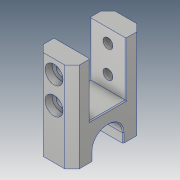
# Autodesk Inventor part: 200-50-WHEEL-CONNECTOR-20MM-01
Saved by Autodesk Inventor 2018.2 (Build 222227000, 227)
## iProperties
Manager: feesmrt
Company: FRANC0R
Created: 2017-12-05
Part Number: 200-50-WHEEL-CONNECTOR-20MM-01
Material: Aluminium 6061
Document SubType Name: Modeling
Designer: feesmrt
Density: 2.7 g/cm^3
Appearance: Aluminium - flach
Project: Rescue Robot
Cost Center: -
Engineer: feesmrt
Authority: feesmrt
Description: Wheel Connector 20mm Part 1
Stock Number: 200-50-WHEEL-CONNECTOR-20MM-01
Author: feesmrt
Subject: Rescue Robot
Title: Wheel Connector 20mm Part 1
Revision Number: 1
Autodesk Inventor part; units mm, degrees
note: some values were not read from the file. Chosen so that the rebuilt part matches the saved one: direction of "DIN7984_M5_Boh".
ref_plane "YZ Plane" through (0, 0, 0) normal (1, 0, 0) x (0, 1, 0)
ref_plane "XZ Plane" through (0, 0, 0) normal (0, 1, 0) x (-1, 0, 0)
ref_plane "XY Plane" through (0, 0, 0) normal (0, 0, 1) x (1, 0, 0)
sketch "Skizze1" plane through (0, 0, 0) normal (1, 0, 0) x (0, 1, 0)
  line L0 (-28, 0) -> (28, 0) construction
  line L1 (0, 35) -> (0, -35) construction
  line L2 (-20, -25) -> (20, -25)
  line L3 (20, -25) -> (20, 25)
  line L4 (20, 25) -> (-20, 25)
  line L5 (-20, 25) -> (-20, -25)
  line L6 (-20, -25) -> (20, 25) construction
  line L7 (20, -25) -> (-20, 25) construction
  point P0 (0, 0)
  dimension "d0" = 40
  dimension "d1" = 50
  constraints: 12 end point, 2 midpoint, 2 parallel, 1 horizontal, 1 perpendicular
  measures "d0" distance of L3.end L4.end
  measures "d1" distance of L2.end L3.end
extrude "Grundkörper" add sketch "Skizze1" along normal mid plane 20
sketch "Skizze2" plane through (10, 0, 0) normal (1, 0, 0) x (0, 0, -1)
  line L0 (-25, 20) -> (-25, -20) construction
  line L1 (0, -28) -> (0, 28) construction
  line L2 (-35, 0) -> (35, 0) construction
  line L3 (-25, -10) -> (5, -10)
  line L4 (5, -10) -> (5, 10)
  line L5 (5, 10) -> (-25, 10)
  line L6 (-25, 10) -> (-25, -10)
  line L7 (25, -20) -> (25, 20) construction
  line L8 (25, -8.4) -> (20, -8.4)
  line L9 (12, -0.4) -> (12, 0.4)
  line L10 (20, 8.4) -> (25, 8.4)
  line L11 (25, -8.4) -> (25, 8.4)
  arc A0 (12, -0.4) -> (20, -8.4) centre (20, -0.4) ccw
  arc A1 (20, 8.4) -> (12, 0.4) centre (20, 0.4) ccw
  point P0 (0, 0)
  dimension "d4" = 30
  dimension "d5" = 20
  dimension "d14" = 13
  dimension "d15" = 16.8
  dimension "d16" = 8
  constraints: 16 end point, 4 perpendicular, 4 point on circle, 4 tangent, 3 point on line, 2 centre point, 2 horizontal, 2 parallel, 1 equal radius, 2 other
  measures "d4" distance of L3.start L3.end
  measures "d5" distance between parallel lines of L5 L3
  measures "d14" distance between parallel lines of L7 L9
  measures "d15" distance between parallel lines of L8 L10
  measures "d16" radius of A0
extrude "Ausschnitt" cut sketch "Skizze2" against normal through all
sketch "Skizze4" plane through (-10, -20, -25) normal (0, -1, 0) x (1, 0, 0)
  line L0 (20, 20) -> (0, 20) construction
  line L1 (20, 50) -> (0, 50) construction
  line L2 (10, 60) -> (10, -10) projected
  line L3 (0, 35) -> (20, 35) construction
  line L4 (0, 0) -> (0, 50) construction
  line L5 (20, 50) -> (20, 0) construction
  point P0 (10, 25)
  point P1 (10, 42.5)
  point P2 (10, 27.5)
  dimension "d19" = 30
  dimension "d20" = 15
  dimension "d21" = 15
  constraints: 4 point on line, 2 end point, 1 horizontal, 1 symmetric about line
  measures "d19" distance between parallel lines of L0 L1
  measures "d20" distance between parallel lines of L1 L3
  measures "d21" distance of point (10, 27.5) point (10, 42.5)
hole "DIN7984_M5_Boh" at (0, -20, 17.5) at (0, -20, 2.5) direction (0, 1, 0) diameter 5.5 end up to surface counterbore diameter 10 counterbore depth 3.9
mirror "Spiegeln_DIN7984_M5_Boh" about plane through (0, 0, 0) normal (0, 1, 0) of "DIN7984_M5_Boh"
sketch "Skizze5" plane through (10, -20, -25) normal (0, 0, -1) x (-1, 0, 0)
  line L0 (0, 0) -> (20, 0) construction
  line L1 (20, 11.6) -> (0, 11.6) construction
  line L2 (20, 40) -> (0, 40) construction
  line L3 (0, 28.4) -> (20, 28.4) construction
  line L4 (10, -8) -> (10, 48) construction
  line L5 (-4, 20) -> (24, 20) construction
  line L6 (10, 11.6) -> (10, 0) construction
  point P0 (10, 20)
  point P1 (10, 5.8)
  point P2 (10, 34.2)
  dimension "d29" = 28.4
  constraints: 3 midpoint, 2 end point, 2 point on line, 1 symmetric about line
  measures "d29" distance of point (10, 34.2) point (10, 5.8)
hole "M5x10" at (0, -14.2, -25) at (0, 14.2, -25) direction (0, 0, 1) diameter 4.134 depth 14.2 tip angle 118 countersink diameter 5 countersink angle 90 thread size "M5x0.8" class "6H" standard "ISO Metric profile"
sketch "Skizze" plane through (10, -20, -25) normal (0, 0, -1) x (-1, 0, 0)
  circle A0 centre (10, 5.8) radius 2.5 projected
  line L0 (20, 11.6) -> (0, 11.6) projected
  line L1 (0, 0) -> (0, 11.6) projected
  line L2 (0, 0) -> (20, 0) projected
  line L3 (20, 11.6) -> (20, 0) projected
  circle A1 centre (10, 34.2) radius 2.5 projected
  line L4 (0, 28.4) -> (20, 28.4) projected
  line L5 (20, 40) -> (20, 28.4) projected
  line L6 (20, 40) -> (0, 40) projected
  line L7 (0, 28.4) -> (0, 40) projected
  line L8 (0, 11.6) -> (0, 19.6) projected
  line L9 (0, 19.6) -> (0, 20.4) projected
  line L10 (0, 20.4) -> (0, 28.4) projected
  line L11 (20, 28.4) -> (20, 20.4) projected
  line L12 (20, 20.4) -> (20, 19.6) projected
  line L13 (20, 19.6) -> (20, 11.6) projected
  point P0 (10, 20)
chamfer "Fase_Allgemein" distance 4 angle 45 4 edges at (10, -20, 0) (-10, -20, 0) (10, 20, 0) (-10, 20, 0)
chamfer "Fase" distance 0.5 angle 45 15 edges at (10, -6.0569, -14.3431) (10, 0, -12) (10, 6.0569, -14.3431) (10, 8.4, -22.5) (10, -8.4, -22.5) (-10, 6.0569, -14.3431) (-10, 0, -12) (-10, -6.0569, -14.3431) (-10, -8.4, -22.5) (-10, 8.4, -22.5) (-10, 0, -5) (-10, 10, 10) (10, -10, 10) (10, 0, -5) (10, 10, 10)
equation "\"d20\" = 0.5 * d19"
equation "\"d21\" = 0.5 * d19"
